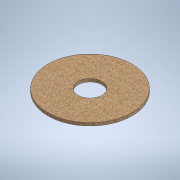
# Autodesk Inventor part: Anillo de Empuje
Saved by Autodesk Inventor 2020 (Build 240168000, 168)
## iProperties
Created: 2021-09-30
Part Number: Anillo de Empuje
Material: MDF Medium Density Fiberboard
Document SubType Name: Modeling
Designer: Carlos
Density: 0.8 g/cm^3
Appearance: Cardboard - Corrugated
Mass: 7.13724 g
Surface Area: 78.4755 cm^2
Volume: 8.92155 cm^3
Author: Carlos
Autodesk Inventor part; units mm, degrees
ref_plane "YZ Plane" through (0, 0, 0) normal (1, 0, 0) x (0, 1, 0)
ref_plane "XZ Plane" through (0, 0, 0) normal (0, 1, 0) x (-1, 0, 0)
ref_plane "XY Plane" through (0, 0, 0) normal (0, 0, 1) x (1, 0, 0)
sketch "Sketch1" plane through (0, 0, 0) normal (0, 1, 0) x (-1, 0, 0)
  circle A0 centre (0, 0) radius 35.17
  circle A1 centre (0, 0) radius 10.05
  dimension "d0" = 70.34
  dimension "d1" = 20.1
  constraints: 2 centre point, 2 coincident
  measures "d0" diameter of A0
  measures "d1" diameter of A1
extrude "Extrusion1" add sketch "Sketch1" along normal blind 2.5
body "Solid1"
